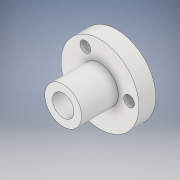
# Autodesk Inventor part: AA038
Saved by Autodesk Inventor 2017 SP1 (Build 210196100, 196)
## iProperties
Created: 2018-01-10
Part Number: AA038
Material: ABS Plastic
Document SubType Name: Modeling
Designer: Zach
Density: 1.06 g/cm^3
Appearance: CR White
Author: Zach
Autodesk Inventor part; units mm, degrees
ref_plane "YZ Plane" through (0, 0, 0) normal (1, 0, 0) x (0, 1, 0)
ref_plane "XZ Plane" through (0, 0, 0) normal (0, 1, 0) x (-1, 0, 0)
ref_plane "XY Plane" through (0, 0, 0) normal (0, 0, 1) x (1, 0, 0)
sketch "Sketch1" plane through (0, 0, 0) normal (0, 0, 1) x (1, 0, 0)
  circle A0 centre (0, 0) radius 7.25
  circle A1 centre (0, 0) radius 12.7
  circle A2 centre (0, 0) radius 9.525 construction
  circle A3 centre (9.525, 0) radius 1.75
  circle A4 centre (-4.7625, 8.2489) radius 1.75
  circle A5 centre (-4.7625, -8.2489) radius 1.75
  dimension "d2" = 19.05
  dimension "d0" = 14.5
  dimension "d1" = 25.4
  dimension "d3" = 3.5
  dimension "d6" = 360
  constraints: 5 centre point, 3 coincident, 2 horizontal alignment, 9 other
  measures "d0" diameter of A0
  measures "d1" diameter of A1
  measures "d3" diameter of A3
extrude "Extrusion1" add sketch "Sketch1" along normal blind 4.5
sketch "Sketch2" plane through (0, 0, 4.5) normal (0, 0, 1) x (1, 0, 0)
  circle A0 centre (0, 0) radius 12.7 projected
  circle A1 centre (-4.7625, 8.2489) radius 1.75 projected
  circle A2 centre (9.525, 0) radius 1.75 projected
  circle A3 centre (-4.7625, -8.2489) radius 1.75 projected
extrude "Extrusion2" add sketch "Sketch2" along normal blind 1
sketch "Sketch3" plane through (0, 0, 5.5) normal (0, 0, 1) x (1, 0, 0)
  line L0 (-4, 0.5) -> (4, 0.5)
  line L1 (4, 0.5) -> (4, -0.5)
  line L2 (4, -0.5) -> (-4, -0.5)
  line L3 (-4, -0.5) -> (-4, 0.5)
  point P0 (0, 0)
  point P1 (4, 0)
  point P2 (0, 0.5)
  dimension "d12" = 1
  dimension "d13" = 8
  constraints: 8 end point, 2 midpoint, 2 parallel, 1 horizontal, 1 horizontal alignment, 1 perpendicular, 1 vertical alignment
  measures "d12" distance of L0.end L1.end
  measures "d13" distance of L0.start L0.end
extrude "Extrusion3" add sketch "Sketch3" along normal blind 1.5
sketch "Sketch4" plane through (0, 0, 5.5) normal (0, 0, 1) x (1, 0, 0)
  circle A0 centre (0, 0) radius 3.5
  circle A1 centre (0, 0) radius 6
  dimension "d16" = 7
  dimension "d17" = 12
  constraints: 2 centre point, 2 coincident
  measures "d16" diameter of A0
  measures "d17" diameter of A1
extrude "Extrusion4" add sketch "Sketch4" along normal blind 12
body "Solid1"
